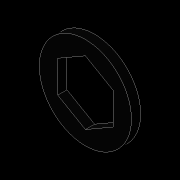
# Autodesk Inventor part: Spacer_0.375hex_0.0625
Saved by Autodesk Inventor 2016 (Build 200138000, 138)
## iProperties
Created: 2015-11-16
Part Number: Spacer_0.375hex_0.0625
Material: Acetal Resin, Black
Document SubType Name: Modeling
Designer: Beezy
Mass: 0.360111 g
Surface Area: 4.85502 cm^2
Volume: 0.252709 cm^3
Density: 1.425 g/cm^3
Appearance: Smooth - Black
Author: Beezy
Autodesk Inventor part; units mm, degrees
ref_plane "YZ Plane" through (0, 0, 0) normal (1, 0, 0) x (0, 1, 0)
ref_plane "XZ Plane" through (0, 0, 0) normal (0, 1, 0) x (-1, 0, 0)
ref_plane "XY Plane" through (0, 0, 0) normal (0, 0, 1) x (1, 0, 0)
sketch "Sketch1" plane through (0, 0, 0) normal (0, 0, 1) x (1, 0, 0)
  circle A0 centre (0, 0) radius 7.9375
  line L0 (0, 5.4993) -> (4.7625, 2.7496)
  line L1 (4.7625, 2.7496) -> (4.7625, -2.7496)
  line L2 (4.7625, -2.7496) -> (0, -5.4993)
  line L3 (0, -5.4993) -> (-4.7625, -2.7496)
  line L4 (-4.7625, -2.7496) -> (-4.7625, 2.7496)
  line L5 (-4.7625, 2.7496) -> (0, 5.4993)
  dimension "d0" = 9.525
  dimension "d1" = 15.875
  constraints: 12 end point, 2 coincident, 1 centre point, 13 other
  measures "d0" distance between parallel lines of L1 L4
  measures "d1" diameter of A0
extrude "Extrusion1" add sketch "Sketch1" along normal blind 1.5875
body "Solid1"
